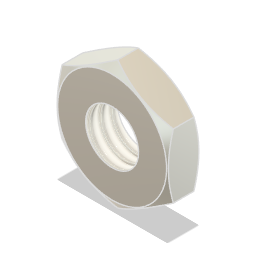
Boreas - RHP02 v14 (Autodesk Fusion 360 archive; units mm, degrees)
design "Hexagon Nut BS 4183 - M4 Steel 6 Plain"
description: Hexagon Nut BS 4183 - M4
part number: HN BS 4183 - M4 Steel 6 Plain
Autodesk Fusion 360 part; units mm, degrees
sketch "Sketch1" plane through (0, 0, 0) normal (0, 1, 0) x (1, 0, 0)
  line L0 (0, 0) -> (0, -2)
  line L1 (-2, 0) -> (-3.43, 0)
  line L2 (-3.43, 0) -> (-4.0425, -0.3536)
  line L3 (-4.0425, -0.3536) -> (-4.0425, -1.6464)
  line L4 (-4.0425, -1.6464) -> (-3.43, -2)
  line L5 (-3.43, -2) -> (-2, -2)
  line L6 (-2, -2) -> (-2, 0)
  dimension "d121" = 4
  dimension "d122" = 30
  dimension "d123" = 30
  dimension "d125" = 6.86
  dimension "d128" = 8.085
  dimension "d152" = 2
  constraint vertical L0
  constraint coincident L0 L0.end
  constraint coincident origin L0
  constraint horizontal L1
  constraint perpendicular L1 L3
  constraint perpendicular L3 L5
  constraint perpendicular L5 L6
  constraint coincident L0.start L1
  constraint coincident L0.start origin
  constraint vertical L1.end L4.end
  constraint coincident L0.end L5
  measures "d122" angle of L1 L2
  measures "d123" angle of L4 L5
  measures "d152" distance of L1.start L5
revolve "Revolve1" add sketch "Sketch1" angle 360 about axis through (0, 0, 0) along (0, 0, 1)
sketch "Sketch8" plane through (0, 0, 2) normal (0, 0, 1) x (1, 0, 0)
  line L0 (0, 0) -> (-7, 0) construction
  line L1 (-3.5, -2.0228) -> (-3.5, 2.0228)
  circle A0 centre (0, 0) radius 2
  circle A1 centre (0, 0) radius 4.0425
  dimension "d114" = 3.5
  constraint horizontal L0
  constraint perpendicular L0 L1
  constraint midpoint L0 L1
  constraint coincident L0.start A0.centre
  constraint coincident L1.end A1
  measures "d114" distance of L0.start L1
extrude "Extrude5" cut sketch "Sketch8" against normal blind 2 contours L1 A1 picked at (-3.5875, -0.4927)
pattern_circular "C-Pattern2" count 6 over 360 about axis through (0, 0, 1.75) along (0, 0, 1) of "Extrude5"
thread "Thread3" "ISO Metric profile 4.0 M4x0.7 M4x0.7 6H" major diameter 4.1095 minor diameter 3.332 pitch 0.7 angle 60 resizes the face on face at (-1.9901, 0.1991, 1.3333)
equation "adsk_nheig = 2.00 mm"
equation "adsk_maxdia = 8.085 mm"
equation "adsk_nomdia = 4.00 mm"
equation "d89 = -adsk_nheig"
equation "adsk_waflat = 7.00 mm"
equation "d114 = adsk_waflat / 2"
equation "adsk_chamang1 = 30 deg"
equation "adsk_chamang2 = 30 deg"
equation "d121 = adsk_nomdia"
equation "d122 = adsk_chamang1"
equation "d123 = adsk_chamang2"
equation "d125 = adsk_beardia"
equation "d128 = adsk_maxdia"
equation "d147 = adsk_nheig"
equation "adsk_beardia = adsk_waflat * 0.98"
equation "d152 = adsk_nheig"
